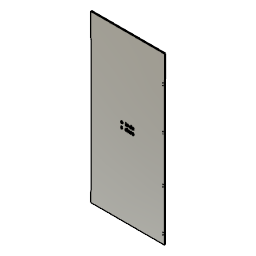
stile_3X82 (Autodesk Fusion 360 design; units mm, degrees)
part number: Configuration 1
Autodesk Fusion 360 part; units mm, degrees
note: some values were not read from the file. Chosen so that the rebuilt part matches the saved one: which bodies a step acts on.
sketch "MasterSketch" plane through (0, 0, 0) normal (0, 1, 0) x (1, 0, 0)
  line L0 (-635, -2870.2) -> (635, -2870.2)
  line L1 (635, -2870.2) -> (635, -25.4)
  line L2 (635, -25.4) -> (-635, -25.4)
  line L3 (-635, -25.4) -> (-635, -2870.2)
  line L4 (0, -25.4) -> (0, 0) construction
  line L5 (602.7928, -2870.2) -> (602.7928, -25.4) construction
  circle A0 centre (602.7928, -2420.112) radius 6.35
  circle A1 centre (602.7928, -2382.012) radius 6.35
  circle A2 centre (602.7928, -161.0995) radius 6.35
  circle A3 centre (602.7928, -199.1995) radius 6.35
  circle A4 centre (602.7928, -1659.1725) radius 6.35
  circle A5 centre (602.7928, -1697.2725) radius 6.35
  circle A6 centre (602.7928, -874.4141) radius 6.35
  circle A7 centre (602.7928, -912.5141) radius 6.35
  circle A8 centre (-602.7928, -2356.612) radius 6.35
  circle A9 centre (-602.7928, -2394.712) radius 6.35
  circle A10 centre (-602.7928, -1661.0436) radius 6.35
  circle A11 centre (-602.7928, -1699.1436) radius 6.35
  circle A12 centre (-602.7928, -966.2689) radius 6.35
  circle A13 centre (-602.7928, -280.2255) radius 6.35
  circle A14 centre (-602.7928, -318.3255) radius 6.35
  line L6 (-602.7928, -2870.2) -> (-602.7928, -25.4) construction
  circle A15 centre (-602.7928, -1004.3689) radius 6.35
  line L7 (-635, -2473.6044) -> (-635, -193.3956)
  arc A16 (-627.38, -222.2445) -> (-635, -193.3956) centre (-685.8, -222.2445) ccw
  line L8 (-627.38, -25.4) -> (-627.38, -2870.2)
  line L9 (-627.38, -1333.5) -> (-635, -1333.5) construction
  arc A17 (-635, -2473.6044) -> (-627.38, -2444.7555) centre (-685.8, -2444.7555) ccw
  line L10 (0, -2870.2) -> (0, 0) construction
  line L11 (0, -228.6) -> (-635, -228.6) construction
  line L12 (-635, -228.6) -> (-762, -228.6) construction
  line L13 (-635, -2438.4) -> (-762, -2438.4) construction
  arc A18 (635, -76.2) -> (627.38, -105.0489) centre (685.8, -105.0489) ccw
  line L14 (627.38, -25.4) -> (627.38, -2870.2)
  line L15 (627.38, -1287.6022) -> (635, -1287.6022) construction
  arc A19 (627.38, -2470.1555) -> (635, -2499.0044) centre (685.8, -2470.1555) ccw
  line L16 (0, -114.3) -> (635, -114.3) construction
  dimension "d10" = 25.4
  dimension "d11" = 2844.8
  dimension "d12" = 1270
  dimension "d24" = 6.35
  dimension "d27" = 6.35
  dimension "d30" = 6.35
  dimension "d32" = 6.35
  dimension "d117" = 6.35
  dimension "d118" = 6.35
  dimension "d119" = 6.35
  dimension "d120" = 6.35
  dimension "d122" = 32.2072
  dimension "d123" = 32.2072
  dimension "d125" = 58.42
  dimension "d137" = 7.62
  dimension "d139" = 396.5956
  dimension "d144" = 228.6
  dimension "d145" = 475.488
  dimension "d146" = 513.588
  dimension "d147" = 1171.0564
  dimension "d148" = 1209.1564
  dimension "d149" = 1865.8311
  dimension "d150" = 1903.9311
  dimension "d151" = 2551.8745
  dimension "d152" = 2589.9745
  dimension "d154" = 228.6
  dimension "d155" = 127
  dimension "d156" = 127
  dimension "d157" = 2209.8
  dimension "d158" = 35.2044
  dimension "d159" = 43.688
  dimension "d160" = 431.8
  dimension "d161" = 51.6255
  dimension "d163" = 7.62
  dimension "d164" = 58.42
  dimension "d184" = 371.1956
  dimension "d185" = 450.088
  dimension "d186" = 488.188
  dimension "d187" = 1172.9276
  dimension "d188" = 1211.0276
  dimension "d189" = 1957.686
  dimension "d190" = 1995.786
  dimension "d191" = 2671.0005
  dimension "d192" = 2709.1005
  dimension "d194" = 114.3
  dimension "d258" = 2794
  dimension "d259" = 2676.8044
  constraint horizontal L0
  constraint vertical L1
  constraint horizontal L2
  constraint vertical L3
  constraint midpoint L2 L4.start
  constraint coincident L4.end L10.end
  constraint vertical L4
  constraint coincident L0 L5.start
  constraint coincident L2 L5.end
  constraint perpendicular L2 L5
  constraint coincident L5 A0.centre
  constraint coincident L5 A1.centre
  constraint equal A0 A1
  constraint equal A2 A3
  constraint coincident L5 A3.centre
  constraint coincident L5 A2.centre
  constraint equal A4 A5
  constraint equal A6 A7
  constraint coincident L5 A5.centre
  constraint coincident L5 A4.centre
  constraint coincident L5 A7.centre
  constraint coincident L5 A6.centre
  constraint coincident A9.centre L6
  constraint coincident A8.centre L6
  constraint equal A8 A9
  constraint equal A13 A14
  constraint coincident A14.centre L6
  constraint coincident A13.centre L6
  constraint equal A10 A11
  constraint equal A12 A15
  constraint coincident A11.centre L6
  constraint coincident A10.centre L6
  constraint coincident A15.centre L6
  constraint coincident A12.centre L6
  constraint coincident L0 L6.start
  constraint coincident L2 L6.end
  constraint vertical L7
  constraint vertical L8
  constraint tangent A16 L8
  constraint coincident L7 L9.end
  constraint perpendicular L7 L9
  constraint symmetric L7.end L9 L7.start
  constraint symmetric A16.start L9 A17.end
  constraint symmetric A16 L9 A17
  constraint collinear L3 L7
  constraint midpoint L0 L10.start
  constraint coincident L0 L8.end
  constraint coincident L8 L9.start
  constraint coincident L2 L8.start
  constraint coincident A16.start L8
  constraint coincident L10 L11.start
  constraint perpendicular L7 L11
  constraint coincident L3 L11.end
  constraint perpendicular L3 L12
  constraint coincident L7 L13.start
  constraint perpendicular L7 L13
  constraint coincident L14 L15.start
  constraint coincident L1 L15.end
  constraint perpendicular L1 L15
  constraint vertical L14
  constraint tangent A18 L14
  constraint coincident A18.end L14
  constraint coincident L1 A18.start
  constraint coincident L2 L14.start
  constraint symmetric A18.end L15 A19.start
  constraint symmetric A18.start L15 A19.end
  constraint symmetric A18 L15 A19
  constraint coincident L7.start A17.start
  constraint coincident L0 L14.end
  constraint coincident L10 L16.start
  constraint coincident L1 L16.end
  constraint perpendicular L1 L16
  measures "d10" distance of L4.start L4.end
  measures "d11" distance of L0.start L2.end
  measures "d12" distance of L1.end L2.end
  measures "d24" radius of A0
  measures "d27" radius of A3
  measures "d30" radius of A5
  measures "d32" radius of A7
  measures "d117" radius of A9
  measures "d118" radius of A14
  measures "d119" radius of A11
  measures "d120" radius of A15
  measures "d122" distance of L1 L5
  measures "d123" distance of L3 L6
  measures "d125" radius of A16
  measures "d137" distance of L3 L8
  measures "d139" distance of L0 L7.start
  measures "d144" distance of L4.end L11
  measures "d145" distance of L0 A9.centre
  measures "d146" distance of L0 A8.centre
  measures "d147" distance of L0 A11.centre
  measures "d148" distance of L0 A10.centre
  measures "d149" distance of L0 A15.centre
  measures "d150" distance of L0 A12.centre
  measures "d151" distance of L0 A14.centre
  measures "d152" distance of L0 A13.centre
  measures "d154" distance of L4.end L12
  measures "d155" distance of L11.end L12.end
  measures "d156" distance of L13.start L13.end
  measures "d157" distance of L12 L13
  measures "d158" distance of L7.start L13
  measures "d159" distance of A9.centre L13
  measures "d160" distance of L0 L13
  measures "d161" distance of A13.centre L11
  measures "d163" distance of L1 L14
  measures "d164" radius of A18
  measures "d184" distance of L0.end A19.end
  measures "d185" distance of L0 A0.centre
  measures "d186" distance of L0 A1.centre
  measures "d187" distance of L0 A5.centre
  measures "d188" distance of L0 A4.centre
  measures "d189" distance of L0 A7.centre
  measures "d190" distance of L0 A6.centre
  measures "d191" distance of L0 A3.centre
  measures "d192" distance of L0 A2.centre
  measures "d194" distance of L4.end L16
  measures "d258" distance of L0 A18.start
  measures "d259" distance of L0 L7.end
extrude "door_extrude" add sketch "MasterSketch" along normal mid plane 19.05 contours L0 L3 L8 A17 | L0 L2 L8 L14 | L3 L7 A16 L8 A17 | L0 L1 L14 A19 | L2 L3 A16 L8 | L1 A18 L14 A19 | L1 L2 A18 L14 | A0 | A1 | A2 | A3 | A4 | A5 | A6 | A7 | A8 | A9 | A10 | A11 | A12 | A13 | A14 | A15 makes body 1 in component "door_panel"
extrude "routing_Left" add sketch "MasterSketch" along normal mid plane 12.7 from surface at -3.175 separate body contours L3 L7 A16 L8 A17 makes body 2 in component "door_panel"
extrude "Extrude6" add sketch "MasterSketch" along normal mid plane 12.7 from surface at 3.175 separate body contours L1 A18 L14 A19 makes body 3 in component "door_panel"
extrude "LR_top_routing" add sketch "MasterSketch" along normal mid plane 12.7 from surface at 19.05 separate body contours L0 L3 L8 A17 makes body 4 in component "door_panel"
extrude "LD_routing_bottom" add sketch "MasterSketch" along normal mid plane 12.7 from surface at 19.05 separate body contours L2 L3 A16 L8 makes body 5 in component "door_panel"
extrude "RD_routing_top" add sketch "MasterSketch" along normal mid plane 12.7 from surface at 19.05 separate body contours L0 L1 L14 A19 makes body 6 in component "door_panel"
extrude "RD_routing_bottom" add sketch "MasterSketch" along normal mid plane 12.7 from surface at 3.175 separate body contours L1 L2 A18 L14 makes body 7 in component "door_panel"
combine "Combine2" operation cut target body 1 tool bodies 3 2 5 7 6 4 in component "door_panel"
extrude "hinge_holes_right" add sketch "MasterSketch" along normal mid plane 14.2875 from surface at 2.3813 separate body contours A0 | A1 | A2 | A3 | A4 | A5 | A6 | A7 makes body 8 at (608.3695, 4.7625, 871.3771) makes body 9 at (609.0169, 4.7625, 2380.7538) makes body 10 at (606.9945, 7.1438, 1692.5113) makes body 11 at (602.6345, 7.1438, 192.8515) makes body 12 at (608.3695, 4.7625, 909.4771) makes body 13 at (609.0169, 4.7625, 2418.8538) makes body 14 at (606.9945, 7.1438, 1654.4113) makes body 15 at (602.6345, 7.1438, 154.7515) in component "door_panel"
extrude "hinge_holes_left" add sketch "MasterSketch" along normal mid plane 14.2875 from surface at 19.05 separate body contours A8 | A9 | A10 | A11 | A12 | A13 | A14 | A15 makes body 16 at (-597.2161, 23.8125, 963.232) makes body 17 at (-596.6392, 23.8125, 2355.0451) makes body 18 at (-598.5911, 23.8125, 1694.3825) makes body 19 at (-602.9511, 23.8125, 311.9775) makes body 20 at (-597.2161, 23.8125, 1001.332) makes body 21 at (-596.6392, 23.8125, 2393.1451) makes body 22 at (-598.5911, 23.8125, 1656.2825) makes body 23 at (-602.9511, 23.8125, 273.8775) in component "door_panel"
combine "Combine3" operation cut target body 1 tool bodies 13 9 10 14 12 8 11 15 19 23 20 16 22 18 21 17 in component "door_panel"
sketch "Labels" plane through (0, 0, 0) normal (0, 1, 0) x (1, 0, 0)
  line L0 (635, -25.4) -> (-635, -2870.2) construction
  line L1 (635, -2870.2) -> (-635, -25.4) construction
  line L2 (139.7, -1371.6) -> (-139.7, -1524) construction
  line L3 (-139.7, -1371.6) -> (139.7, -1371.6) construction
  line L4 (139.7, -1371.6) -> (139.7, -1524) construction
  line L5 (139.7, -1524) -> (-139.7, -1524) construction
  line L6 (-139.7, -1524) -> (-139.7, -1371.6) construction
  point P0 (-635, -2870.2)
  point P1 (635, -2870.2)
  point P2 (635, -25.4)
  point P3 (-635, -25.4)
  point P4 (0, -1447.8)
  dimension "d78" = 50.8
  dimension "d220" = 279.4
  dimension "d221" = 152.4
  text T0 "outside surface" font "Arial" height 50.8 align centre top in box 279.4 x 152.4 at (-139.7, -1371.6) x (1, 0) y (0, -1) spacing 1
  constraint coincident P2 L0.start
  constraint coincident P0 L0.end
  constraint coincident P1 L1.start
  constraint coincident P3 L1.end
  constraint coincident L0 P4
  constraint coincident L1 P4
  constraint midpoint P4 L2
  constraint horizontal L5
  constraint coincident L2.start
  constraint coincident L2.end
extrude "Extrude1" add sketch "Labels" against normal blind 3.175 from surface at -12.7 separate body text T0 makes body 24 at (49.5025, -12.7, 1401.1814) makes body 25 at (-34.3402, -12.7, 1412.605) makes body 26 at (-94.3116, -12.7, 1412.8762) makes body 27 at (100.4911, -12.7, 1491.7158) makes body 28 at (26.89, -12.7, 1497.7337) makes body 29 at (6.2835, -12.7, 1492.1603) makes body 30 at (-42.2756, -12.7, 1491.1613) makes body 31 at (-25.1459, -12.7, 1490.9188) makes body 32 at (26.89, -12.7, 1521.609) makes body 33 at (68.2455, -12.7, 1497.3881) makes body 34 at (-109.358, -12.7, 1494.1432) makes body 35 at (-48.2011, -12.7, 1411.8773) makes body 36 at (34.662, -12.7, 1404.3629) makes body 37 at (102.4317, -12.7, 1412.4317) in component "OutLabel"
component "door_panel" placed x (1, 0, 0) y (0, 1, 0) z (0, 0, 1) at (0, 0, 0)
component "OutLabel" placed x (1, 0, 0) y (0, 1, 0) z (0, 0, 1) at (0, 0, 0)
equation "component_height = 112 in" comment "001) Input - Model     Height of the stile"
equation "component_width = 50 in" comment "000) Input - Model     Width of the component in inches"
equation "levelling_gap = 1 in" comment "006) Fixed - Helper     We leave a 1\" gap between the bottom of the stile and the floor to account for anchoring hardware"
equation "d10 = levelling_gap"
equation "d11 = component_height"
equation "d12 = component_width"
equation "hole_radius = 0.25 in" comment "013) Fixed - Model     Radius of drilled holes"
equation "component_thickness = 0.75 in" comment "014) Fixed - Helper     Thickness of the component"
equation "door_top_margin = 1.72 in" comment "004) Fixed - Helper     Distance between top-most hole and top of door"
equation "LD_bottom_margin = 1.72 in + if(LD_floor_clearance == 1 in; door_notching_y_dist; 0 in)" comment "107) Derived - Helper     Distance between bottom-most hole and bottom of door on the door adjacent to the LEFT side of the stile"
equation "LD_swinging_out = 1" comment "103) Input - Helper     For the door adjacent to the LEFT side of the stile: whether it is an outswing door"
equation "hinge_hole_space = 1.5 in" comment "005) Fixed - Helper     Distance between a hinge's tope and bottom hole"
equation "d24 = hole_radius"
equation "d27 = hole_radius"
equation "d30 = hole_radius"
equation "d32 = hole_radius"
equation "hinge_hole_x_dist = 1.268 in" comment "002) Fixed - Model     Horizontal distance between hinge holes and edge of stile"
equation "d39 = component_thickness"
equation "rabbeting_width = 0.3 in" comment "012) Fixed - Model     Width of the rabbeting"
equation "rabbeting_depth = 0.5 in" comment "015) Fixed - Helper     Depth of rabbeting"
equation "d47 = left_rabbeting_activation_offset"
equation "d48 = rabbeting_depth"
equation "hinge_hole_depth = 0.5625 in" comment "016) Fixed - Helper     Depth of hinge hole"
equation "d51 = hinge_hole_depth"
equation "d53 = if(right_exterior_drilling; -component_thickness / 2 + hinge_hole_depth / 2; if(right_interior_drilling; component_thickness / 2 - hinge_hole_depth / 2; component_thickness))"
equation "d79 = 'outside surface'"
equation "d82 = ( 1 / 8 ) * 1 in"
equation "d83 = ( 1 / 8 ) * 1 in"
equation "LD_top_hinge_hole_1_y_value = door_top_margin" comment "121) Derived - Helper     Distance between top of the left door and the center of the door hinge hole"
equation "LD_top_hinge_hole_2_y_value = LD_top_hinge_hole_1_y_value + hinge_hole_space" comment "122) Derived - Helper     Distance between top of the left door and the center of the door hinge hole"
equation "LD_inter_hinge_gap = ( LD_height - ( door_top_margin ) - ( LD_bottom_margin + hinge_hole_space ) ) / 3" comment "106) Derived - Helper     Distance between top_hinge_holes of adjacent hinges on the door adjacent to the LEFT side of the stile"
equation "LD_mid_top_hinge_offset = ( -1 * 0.823 * if(LD_floor_clearance == 1 in; 1; 0) ) * 1 in" comment "108) Derived - Helper     For the door adjacent to the LEFT side of the stile: An offset applying to the mid-top hinge when the floor clearance is 1\" the door hinges on a stile"
equation "LD_mid_top_hinge_hole_1_y_value = LD_top_hinge_hole_1_y_value + LD_inter_hinge_gap + LD_mid_top_hinge_offset" comment "123) Derived - Helper     Distance between top of the left door and the center of the door hinge hole"
equation "LD_mid_top_hinge_hole_2_y_value = LD_mid_top_hinge_hole_1_y_value + hinge_hole_space" comment "124) Derived - Helper     Distance between top of the left door and the center of the door hinge hole"
equation "LD_mid_bottom_hinge_offset = ( 2 * 0.823 * if(LD_floor_clearance == 1 in; 1; 0) ) * 1 in" comment "109) Derived - Helper     For the door adjacent to the LEFT side of the stile: An offset applying to the mid-bottom hinge when the floor clearance is 1\" the door hinges on a stile"
equation "LD_mid_bottom_hinge_hole_1_y_value = LD_mid_top_hinge_hole_1_y_value + LD_inter_hinge_gap + LD_mid_bottom_hinge_offset" comment "125) Derived - Helper     Distance between top of the left door and the center of the door hinge hole"
equation "LD_mid_bottom_hinge_hole_2_y_value = LD_mid_bottom_hinge_hole_1_y_value + hinge_hole_space" comment "126) Derived - Helper     Distance between top of the left door and the center of the door hinge hole"
equation "LD_bottom_hinge_hole_1_y_value = LD_mid_bottom_hinge_hole_1_y_value + LD_inter_hinge_gap + LD_mid_top_hinge_offset" comment "127) Derived - Helper     Distance between top of the left door and the center of the door hinge hole"
equation "LD_bottom_hinge_hole_2_y_value = LD_bottom_hinge_hole_1_y_value + hinge_hole_space" comment "128) Derived - Helper     Distance between top of the left door and the center of the door hinge hole"
equation "left_rabbeting_activation_offset = if(left_interior_rabbeting; ( 1 / 8 ) * 1 in; if(left_exterior_rabbeting; ( -1 / 8 ) * 1 in; component_thickness))" comment "113) Fixed - Helper     An offset that repositions a void relative to the component, allowing the void to cut into the panel at the specified location and create left rabbeting on the model"
equation "right_rabbeting_activation_offset = if(right_interior_rabbeting; ( 1 / 8 ) * 1 in; if(right_exterior_rabbeting; ( -1 / 8 ) * 1 in; component_thickness))" comment "213) Fixed - Helper     An offset that repositions a void relative to the component, allowing the void to cut into the panel at the specified location and create right rabbeting on the model"
equation "d114 = rabbeting_depth"
equation "d116 = right_rabbeting_activation_offset"
equation "d117 = hole_radius"
equation "d118 = hole_radius"
equation "d119 = hole_radius"
equation "d120 = hole_radius"
equation "d122 = hinge_hole_x_dist"
equation "d123 = hinge_hole_x_dist"
equation "LD_floor_clearance = 9 in" comment "105) Input - Helper     Floor clearance of the door adjacent to the LEFT side of the stile (when viewed from outside the stall)"
equation "LD_height = 87 in" comment "104) Input - Helper     Height of the door adjacent to the LEFT side of the stile (when viewed from outside the stall)"
equation "LD_stile_hole_modifier = component_height - ( LD_height + LD_floor_clearance - levelling_gap )" comment "110) Derived - Helper     For the door adjacent to the LEFT side of the stile: Adjustment factor convert door y coordinates to stile y coordinates"
equation "rabbeting_start_above_door = ( ( 0.75 + 2.022 ) / 2 ) * 1 in" comment "010) Fixed - Helper     Distance by which rabbeting extends above door"
equation "rabbeting_stop_below_door = ( ( 0.75 + 2.022 ) / 2 ) * 1 in" comment "011) Fixed - Helper     Distance by which rabbeting extends below door"
equation "d137 = rabbeting_width"
equation "rabbeting_insertion_radius = 2.3 in" comment "017) Fixed - Helper     Radius of the rabbetting insertion curve"
equation "d139 = left_rabbeting_start"
equation "d144 = if(LD_floor_clearance <= 4.5 in; 4.5 in; LD_floor_clearance)"
equation "d145 = LD_stile_top_hinge_hole_1_y_value"
equation "d146 = LD_stile_top_hinge_hole_2_y_value"
equation "d147 = LD_stile_mid_top_hinge_hole_1_y_value"
equation "d148 = LD_stile_mid_top_hinge_hole_2_y_value"
equation "d149 = LD_stile_mid_bottom_hinge_hole_1_y_value"
equation "d150 = LD_stile_mid_bottom_hinge_hole_2_y_value"
equation "d151 = LD_stile_bottom_hinge_hole_1_y_value"
equation "d152 = LD_stile_bottom_hinge_hole_2_y_value"
equation "d154 = LD_floor_clearance"
equation "d157 = LD_height"
equation "d163 = rabbeting_width"
equation "d164 = rabbeting_insertion_radius"
equation "RD_swinging_out = 0" comment "203) Input - Helper     For the door adjacent to the LEFT side of the stile: whether it is an outswing door"
equation "RD_floor_clearance = 1 in" comment "205) Input - Helper     Floor clearance of the door adjacent to the RIGHT side of the stile (when viewed from outside the stall)"
equation "RD_height = 96 in" comment "204) Input - Helper     Height of the door adjacent to the RIGHT side of the stile (when viewed from outside the stall)"
equation "RD_stile_hole_modifier = component_height - ( RD_height + RD_floor_clearance - levelling_gap )" comment "210) Derived - Helper     For the door adjacent to the RIGHT side of the stile: Adjustment factor convert door y coordinates to stile y coordinates"
equation "RD_top_hinge_hole_1_y_value = door_top_margin" comment "221) Derived - Helper     Distance between top of the right door and the center of the door hinge hole"
equation "RD_top_hinge_hole_2_y_value = RD_top_hinge_hole_1_y_value + hinge_hole_space" comment "222) Derived - Helper     Distance between top of the right door and the center of the door hinge hole"
equation "RD_inter_hinge_gap = ( RD_height - ( door_top_margin ) - ( RD_bottom_margin + hinge_hole_space ) ) / 3" comment "206) Derived - Helper     Distance between top_hinge_holes of adjacent hinges on the door adjacent to the RIGHT side of the stile"
equation "RD_mid_top_hinge_offset = ( -1 * 0.823 * if(RD_floor_clearance == 1 in; 1; 0) ) * 1 in" comment "208) Derived - Helper     For the door adjacent to the RIGHT side of the stile: An offset applying to the mid-top hinge when the floor clearance is 1\" the door hinges on a stile"
equation "RD_mid_top_hinge_hole_1_y_value = RD_top_hinge_hole_1_y_value + RD_inter_hinge_gap + RD_mid_top_hinge_offset" comment "223) Derived - Helper     Distance between top of the right door and the center of the door hinge hole"
equation "RD_mid_top_hinge_hole_2_y_value = RD_mid_top_hinge_hole_1_y_value + hinge_hole_space" comment "224) Derived - Helper     Distance between top of the right door and the center of the door hinge hole"
equation "RD_mid_bottom_hinge_offset = ( 2 * 0.823 * if(RD_floor_clearance == 1 in; 1; 0) ) * 1 in" comment "209) Derived - Helper     For the door adjacent to the RIGHT side of the stile: An offset applying to the mid-bottom hinge when the floor clearance is 1\" the door hinges on a stile"
equation "RD_mid_bottom_hinge_hole_1_y_value = RD_mid_top_hinge_hole_1_y_value + RD_inter_hinge_gap + RD_mid_bottom_hinge_offset" comment "225) Derived - Helper     Distance between top of the right door and the center of the door hinge hole"
equation "RD_mid_bottom_hinge_hole_2_y_value = RD_mid_bottom_hinge_hole_1_y_value + hinge_hole_space" comment "226) Derived - Helper     Distance between top of the right door and the center of the door hinge hole"
equation "RD_bottom_hinge_hole_1_y_value = RD_mid_bottom_hinge_hole_1_y_value + RD_inter_hinge_gap + RD_mid_top_hinge_offset" comment "227) Derived - Helper     Distance between top of the right door and the center of the door hinge hole"
equation "RD_bottom_hinge_hole_2_y_value = RD_bottom_hinge_hole_1_y_value + hinge_hole_space" comment "228) Derived - Helper     Distance between top of the right door and the center of the door hinge hole"
equation "d184 = right_rabbeting_start"
equation "d185 = RD_stile_top_hinge_hole_1_y_value"
equation "d186 = RD_stile_top_hinge_hole_2_y_value"
equation "d187 = RD_stile_mid_top_hinge_hole_1_y_value"
equation "d188 = RD_stile_mid_top_hinge_hole_2_y_value"
equation "d189 = RD_stile_mid_bottom_hinge_hole_1_y_value"
equation "d190 = RD_stile_mid_bottom_hinge_hole_2_y_value"
equation "d191 = RD_stile_bottom_hinge_hole_1_y_value"
equation "d192 = RD_stile_bottom_hinge_hole_2_y_value"
equation "d194 = if(RD_floor_clearance <= 4.5 in; 4.5 in; RD_floor_clearance)"
equation "left_side_door = 1" comment "101) Input - Helper     Whether there is a door adjacent to the left side of the stile"
equation "right_side_door = 1" comment "201) Input - Helper     Whether there is a door adjacent to the left side of the stile"
equation "d198 = if(LD_full_rabbeting_top; left_rabbeting_activation_offset; component_thickness)"
equation "d199 = rabbeting_depth"
equation "LD_full_rabbeting_top = if(LD_stile_hole_modifier - rabbeting_start_above_door <= 2 in and left_side_door; 1; 0)" comment "114) Derived - Helper     Whether rabbeting on the stile's left side extends all the way to the top"
equation "RD_full_rabbeting_top = if(RD_stile_hole_modifier - rabbeting_start_above_door <= 2 in and right_side_door; 1; 0)" comment "214) Derived - Helper     Whether rabbeting on the stile's right side extends all the way to the top"
equation "LD_full_rabbeting_bottom = if(LD_floor_clearance <= 4.5 in and left_side_door; 1; 0)" comment "115) Derived - Helper     Whether rabbeting on the stile's left side extends all the way to the bottom"
equation "RD_full_rabbeting_bottom = ( if(RD_floor_clearance <= 4.5 in and right_side_door; 1; 0) )" comment "215) Derived - Helper     Whether rabbeting on the stile's right side extends all the way to the bottom"
equation "d208 = if(LD_full_rabbeting_bottom; left_rabbeting_activation_offset; component_thickness)"
equation "d209 = rabbeting_depth"
equation "d211 = if(RD_full_rabbeting_top; right_rabbeting_activation_offset; component_thickness)"
equation "d212 = rabbeting_depth"
equation "d214 = if(RD_full_rabbeting_bottom; right_rabbeting_activation_offset; component_thickness)"
equation "d215 = rabbeting_depth"
equation "d217 = if(left_exterior_drilling; -component_thickness / 2 + hinge_hole_depth / 2; if(left_interior_drilling; component_thickness / 2 - hinge_hole_depth / 2; component_thickness))"
equation "d218 = hinge_hole_depth"
equation "door_notching_y_dist = 3.31 in" comment "003) Fixed - Helper     Height of notching cutout from bottom of door"
equation "stile_mid_top_hinge_offset = 1 / 32 * in" comment "007) Fixed - Helper     an offset between the position of this hinge on the stile vs the door"
equation "stile_mid_bottom_hinge_offset = ( 1 / 32 ) * 1 in" comment "008) Fixed - Helper     an offset between the position of this hinge on the stile vs the door"
equation "stile_bottom_hinge_offset = ( -5 / 16 ) * 1 in" comment "009) Fixed - Helper     an offset between the position of this hinge on the stile vs the door"
equation "LD_hinging_right = 0" comment "102) Input - Helper     For the door adjacent to the LEFT side of the stile: whether it's hinges are on the right side of the door"
equation "left_interior_rabbeting = if(left_side_door and not(LD_swinging_out); 1; 0)" comment "111) Derived - Model     Whether rabbeting is present the interior left edge of the stile"
equation "left_exterior_rabbeting = if(left_side_door and LD_swinging_out; 1; 0)" comment "112) Derived - Model     Whether rabbeting is present the exterior left edge of the stile"
equation "left_interior_drilling = if(left_side_door and LD_hinging_right and not(LD_swinging_out); 1; 0)" comment "118) Derived - Model     Whether drilling is present the interior left edge of the stile"
equation "left_exterior_drilling = if(left_side_door and LD_hinging_right and LD_swinging_out; 1; 0)" comment "119) Derived - Model     Whether drilling is present the exterior left edge of the stile"
equation "LD_stile_top_hinge_hole_1_y_value = LD_top_hinge_hole_1_y_value + LD_stile_hole_modifier" comment "131) Derived - Model     Distance between top of stile and center of stile's left side hinge hole"
equation "LD_stile_top_hinge_hole_2_y_value = LD_stile_top_hinge_hole_1_y_value + hinge_hole_space" comment "132) Derived - Model     Distance between top of stile and center of stile's left side hinge hole"
equation "LD_stile_mid_top_hinge_hole_1_y_value = LD_mid_top_hinge_hole_1_y_value + LD_stile_hole_modifier + stile_mid_top_hinge_offset" comment "133) Derived - Model     Distance between top of stile and center of stile's left side hinge hole"
equation "LD_stile_mid_top_hinge_hole_2_y_value = LD_stile_mid_top_hinge_hole_1_y_value + hinge_hole_space" comment "134) Derived - Model     Distance between top of stile and center of stile's left side hinge hole"
equation "LD_stile_mid_bottom_hinge_hole_1_y_value = LD_mid_bottom_hinge_hole_1_y_value + LD_stile_hole_modifier + stile_mid_bottom_hinge_offset" comment "135) Derived - Model     Distance between top of stile and center of stile's left side hinge hole"
equation "LD_stile_mid_bottom_hinge_hole_2_y_value = LD_stile_mid_bottom_hinge_hole_1_y_value + hinge_hole_space" comment "136) Derived - Model     Distance between top of stile and center of stile's left side hinge hole"
equation "LD_stile_bottom_hinge_hole_1_y_value = LD_bottom_hinge_hole_1_y_value + LD_stile_hole_modifier + stile_bottom_hinge_offset" comment "137) Derived - Model     Distance between top of stile and center of stile's left side hinge hole"
equation "LD_stile_bottom_hinge_hole_2_y_value = LD_stile_bottom_hinge_hole_1_y_value + hinge_hole_space" comment "138) Derived - Model     Distance between top of stile and center of stile's left side hinge hole"
equation "left_rabbeting_start = if(LD_stile_hole_modifier - rabbeting_start_above_door <= 2 in; 2 in; LD_stile_hole_modifier - rabbeting_start_above_door)" comment "116) Derived - Model     Distance from the top edge of the stile to the beginning of rabbeting on the left side of the stile. if the distance between the door and the top of the still is <2\"\" then the rabbeting starts at the beginning of the stile with no radius cut in."
equation "left_rabbeting_stop = if(LD_floor_clearance <= 4.5 in; component_height - 2 in; LD_stile_hole_modifier + LD_height + rabbeting_stop_below_door)" comment "117) Derived - Model     Distance from the top edge of the stile to the end of rabbeting on the left side of the stile. if the door_floor_clearance equals 1\" or 4.5\", then the rabbeting goes all the way to the end of the stile with no radius cut in."
equation "RD_hinging_right = 1" comment "202) Input - Helper     For the door adjacent to the LEFT side of the stile: whether it's hinges are on the right side of the door"
equation "RD_bottom_margin = 1.72 in + if(RD_floor_clearance == 1 in; door_notching_y_dist; 0 in)" comment "207) Derived - Helper     Distance between bottom-most hole and bottom of door on the door adjacent to the RIGHT side of the stile"
equation "right_interior_rabbeting = if(right_side_door and not(RD_swinging_out); 1; 0)" comment "211) Derived - Model     Whether rabbeting is present the interior right edge of the stile"
equation "right_exterior_rabbeting = if(right_side_door and RD_swinging_out; 1; 0)" comment "212) Derived - Model     Whether rabbeting is present the exterior right edge of the stile"
equation "right_interior_drilling = if(right_side_door and RD_hinging_right and not(RD_swinging_out); 1; 0)" comment "218) Derived - Model     Whether drilling is present the interior right edge of the stile"
equation "right_exterior_drilling = if(right_side_door and RD_hinging_right and RD_swinging_out; 1; 0)" comment "219) Derived - Model     Whether drilling is present the exterior right edge of the stile"
equation "RD_stile_top_hinge_hole_1_y_value = RD_top_hinge_hole_1_y_value + RD_stile_hole_modifier" comment "231) Derived - Model     Distance between top of stile and center of stile's right side hinge hole"
equation "RD_stile_top_hinge_hole_2_y_value = RD_stile_top_hinge_hole_1_y_value + hinge_hole_space" comment "232) Derived - Model     Distance between top of stile and center of stile's right side hinge hole"
equation "RD_stile_mid_top_hinge_hole_1_y_value = RD_mid_top_hinge_hole_1_y_value + RD_stile_hole_modifier + stile_mid_top_hinge_offset" comment "233) Derived - Model     Distance between top of stile and center of stile's right side hinge hole"
equation "RD_stile_mid_top_hinge_hole_2_y_value = RD_stile_mid_top_hinge_hole_1_y_value + hinge_hole_space" comment "234) Derived - Model     Distance between top of stile and center of stile's right side hinge hole"
equation "RD_stile_mid_bottom_hinge_hole_1_y_value = RD_mid_bottom_hinge_hole_1_y_value + RD_stile_hole_modifier + stile_mid_bottom_hinge_offset" comment "235) Derived - Model     Distance between top of stile and center of stile's right side hinge hole"
equation "RD_stile_mid_bottom_hinge_hole_2_y_value = RD_stile_mid_bottom_hinge_hole_1_y_value + hinge_hole_space" comment "236) Derived - Model     Distance between top of stile and center of stile's right side hinge hole"
equation "RD_stile_bottom_hinge_hole_1_y_value = RD_bottom_hinge_hole_1_y_value + RD_stile_hole_modifier + stile_bottom_hinge_offset" comment "237) Derived - Model     Distance between top of stile and center of stile's right side hinge hole"
equation "RD_stile_bottom_hinge_hole_2_y_value = RD_stile_bottom_hinge_hole_1_y_value + hinge_hole_space" comment "238) Derived - Model     Distance between top of stile and center of stile's right side hinge hole"
equation "right_rabbeting_start = if(RD_stile_hole_modifier - rabbeting_start_above_door <= 2 in; 2 in; RD_stile_hole_modifier - rabbeting_start_above_door)" comment "216) Derived - Model     Distance from the top edge of the stile to the beginning of rabbeting on the right side of the stile. if the distance between the door and the top of the still is <2\"\" then the rabbeting starts at the beginning of the stile with no radius cut in."
equation "right_rabbeting_stop = if(RD_floor_clearance <= 4.5 in; component_height - 2 in; RD_stile_hole_modifier + LD_height + rabbeting_stop_below_door)" comment "217) Derived - Model     Distance from the top edge of the stile to the end of rabbeting on the right side of the stile. if the door_floor_clearance equals 1\" or 4.5\", then the rabbeting goes all the way to the end of the stile with no radius cut in."
equation "d258 = right_rabbeting_stop"
equation "d259 = left_rabbeting_stop"
equation "LD_height_limited = min(96 in; max(73 in; LD_height))"
equation "d143 = stile_routing_start_below_door"
equation "LD_floor_clearance_limited = min(12 in; max(1 in; LD_floor_clearance))"
equation "door_notching_y_distance = 3.31 in"
equation "RD_floor_clearance_limited = min(12 in; max(1 in; RD_floor_clearance))"
equation "RD_height_limited = min(96 in; max(73 in; RD_height))"
named bodies: "door_panel", "RightRout"
